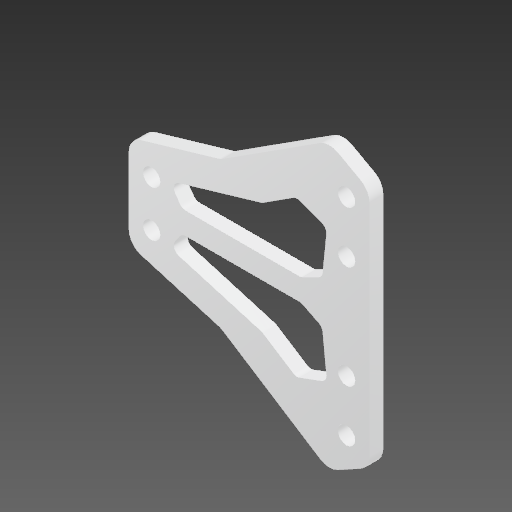
# Autodesk Inventor part: ShoulderBracket
Saved by Autodesk Inventor 2020 (Build 240168000, 168)
## iProperties
Created: 2020-04-01
Part Number: ShoulderBracket
Material: Aluminum 6061
Document SubType Name: Modeling
Designer: valer
Density: 2.7 g/cm^3
Appearance: Aluminum - Flat
Author: valer
Autodesk Inventor part; units mm, degrees
ref_plane "YZ Plane" through (0, 0, 0) normal (1, 0, 0) x (0, 1, 0)
ref_plane "XZ Plane" through (0, 0, 0) normal (0, 1, 0) x (-1, 0, 0)
ref_plane "XY Plane" through (0, 0, 0) normal (0, 0, 1) x (1, 0, 0)
sketch "Base" plane through (0, 0, 0) normal (0, 0, 1) x (1, 0, 0)
  line L0 (0, 0) -> (-88.9, 0) construction
  line L1 (0, 0) -> (0, -44.3545)
  line L2 (-54.8996, -27.0065) -> (-15.0024, -52.5816)
  line L3 (-15.0024, -52.5816) -> (0, -44.3545)
  line L4 (-27.0114, -28.7632) -> (-15.7142, -24.572)
  line L5 (-25.2668, -4.064) -> (-17.4625, -7.9375)
  line L6 (-69.1942, -4.064) -> (-73.825, -10.6243)
  line L7 (-69.1942, -4.064) -> (-25.2668, -4.064)
  line L8 (-73.825, -10.6243) -> (-39.6875, -20.6375)
  line L9 (-17.4625, -7.9375) -> (-15.7142, -24.572)
  line L10 (-39.6875, -20.6375) -> (-27.0114, -28.7632)
  line L11 (-88.9, 0) -> (-88.9, -17.0334)
  line L12 (-88.9, -17.0334) -> (-54.8996, -27.0065)
  line L13 (0, 0) -> (0, 44.3545)
  line L14 (-54.8996, 27.0065) -> (-15.0024, 52.5816)
  line L15 (-15.0024, 52.5816) -> (0, 44.3545)
  line L16 (-27.0114, 28.7632) -> (-15.7142, 24.572)
  line L17 (-25.2668, 4.064) -> (-17.4625, 7.9375)
  line L18 (-69.1942, 4.064) -> (-73.825, 10.6243)
  line L19 (-69.1942, 4.064) -> (-25.2668, 4.064)
  line L20 (-73.825, 10.6243) -> (-39.6875, 20.6375)
  line L21 (-17.4625, 7.9375) -> (-15.7142, 24.572)
  line L22 (-39.6875, 20.6375) -> (-27.0114, 28.7632)
  line L23 (-88.9, 0) -> (-88.9, 17.0334)
  line L24 (-88.9, 17.0334) -> (-54.8996, 27.0065)
  dimension "d39" = 88.9
  dimension "d44" = 4.064
  constraints: 50 end point, 11 symmetric about line, 2 horizontal, 2 parallel, 2 vertical
  measures "d39" distance of L0.start L0.end
  measures "d44" distance between parallel lines of L7 L0
extrude "Extrusion3" add sketch "Base" along normal blind 5.08
fillet "Fillet5" radius 6.35 8 edges at (-15.0024, 52.5816, 2.54) (0, 44.3545, 2.54) (-88.9, 17.0334, 2.54) (-88.9, -17.0334, 2.54) (-54.8996, -27.0065, 2.54) (-15.0024, -52.5816, 2.54) (0, -44.3545, 2.54) (-54.8996, 27.0065, 2.54)
fillet "Fillet6" radius 2.54 14 edges at (-73.825, 10.6243, 2.54) (-73.825, -10.6243, 2.54) (-69.1942, -4.064, 2.54) (-69.1942, 4.064, 2.54) (-39.6875, 20.6375, 2.54) (-27.0114, 28.7632, 2.54) (-15.7142, 24.572, 2.54) (-17.4625, 7.9375, 2.54) (-25.2668, 4.064, 2.54) (-25.2668, -4.064, 2.54) (-17.4625, -7.9375, 2.54) (-15.7142, -24.572, 2.54) (-27.0114, -28.7632, 2.54) (-39.6875, -20.6375, 2.54)
sketch "Sketch6" plane through (0, 0, 5.08) normal (0, 0, 1) x (1, 0, 0)
  line L0 (-106.68, 0) -> (17.78, 0) projected
  line L1 (-8.4667, 0) -> (-8.4667, -38.1) construction
  line L2 (0, -40.5946) -> (0, 40.5946) projected
  circle A0 centre (-8.4667, -19.05) radius 3.175
  circle A1 centre (-8.4667, -38.1) radius 3.175
  circle A2 centre (-80.4333, -8.4667) radius 3.175
  line L3 (-88.9, 12.2785) -> (-88.9, -12.2785) projected
  circle A3 centre (-8.4667, 19.05) radius 3.175
  circle A4 centre (-8.4667, 38.1) radius 3.175
  circle A5 centre (-80.4333, 8.4667) radius 3.175
  point P0 (0, 0)
  dimension "d49" = 8.4667
  dimension "d50" = 38.1
  dimension "d51" = 6.35
  dimension "d53" = 8.4667
  dimension "d54" = 8.4667
  constraints: 6 centre point, 3 symmetric about line, 2 end point, 2 equal radius, 1 coincident, 1 midpoint, 1 point on line, 1 vertical, 3 other
  measures "d49" distance between parallel lines of L2 L1
  measures "d50" distance of L1.start L1.end
  measures "d51" diameter of A0
  measures "d53" distance from line of L0 A2.centre
  measures "d54" distance from line of L3 A2.centre
extrude "Extrusion5" cut sketch "Sketch6" against normal blind 5.08
body "Solid2"
